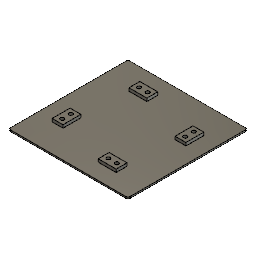
force_plate_bottom (Autodesk Fusion 360 design; units mm, degrees)
Autodesk Fusion 360 part; units mm, degrees
sketch "Sketch1" plane through (0, 0, 0) normal (0, 1, 0) x (1, 0, 0)
  line L0 (-67.5, -70) -> (67.5, -70)
  line L1 (70, -67.5) -> (70, 67.5)
  line L2 (67.5, 70) -> (-67.5, 70)
  line L3 (-70, 67.5) -> (-70, -67.5)
  line L4 (-70, -70) -> (70, 70) construction
  line L5 (70, -70) -> (-70, 70) construction
  arc A0 (-67.5, 70) -> (-70, 67.5) centre (-67.5, 67.5) ccw
  arc A1 (70, 67.5) -> (67.5, 70) centre (67.5, 67.5) ccw
  arc A2 (67.5, -70) -> (70, -67.5) centre (67.5, -67.5) ccw
  arc A3 (-70, -67.5) -> (-67.5, -70) centre (-67.5, -67.5) ccw
  dimension "d1" = 140
  dimension "d2" = 140
  dimension "d25" = 2.5
  dimension "d26" = 2.5
  dimension "d27" = 2.5
  dimension "d28" = 2.5
  constraint horizontal L0
  constraint perpendicular L0 L1
  constraint parallel L0 L2
  constraint parallel L1 L3
  constraint coincident L4 origin
  constraint coincident L5 origin
  constraint coincident L5.end L2
  constraint coincident L5.end L3
  constraint tangent L2 A0
  constraint tangent L3 A0
  constraint coincident L4.end L2
  constraint coincident L4.end L1
  constraint tangent L2 A1
  constraint tangent L1 A1
  constraint coincident L5.start L1
  constraint coincident L5.start L0
  constraint tangent L1 A2
  constraint tangent L0 A2
  constraint coincident L4.start L3
  constraint coincident L4.start L0
  constraint tangent L3 A3
  constraint tangent L0 A3
  measures "d1" distance of L4.end L5.end
  measures "d2" distance of L5.start L4.end
  measures "d25" radius of A0
  measures "d26" radius of A1
  measures "d27" radius of A2
  measures "d28" radius of A3
extrude "Extrude1" add sketch "Sketch1" along normal blind 2
sketch "Sketch11" plane through (0, 0, 0) normal (0, -1, 0) x (1, 0, 0)
  arc A0 (-67.5, 70) -> (-70, 67.5) centre (-67.5, 67.5) ccw
  line L0 (-70, 67.5) -> (-70, -67.5)
  arc A1 (-70, -67.5) -> (-67.5, -70) centre (-67.5, -67.5) ccw
  line L1 (-67.5, -70) -> (67.5, -70)
  arc A2 (67.5, -70) -> (70, -67.5) centre (67.5, -67.5) ccw
  line L2 (70, -67.5) -> (70, 67.5)
  arc A3 (70, 67.5) -> (67.5, 70) centre (67.5, 67.5) ccw
  line L3 (67.5, 70) -> (-67.5, 70)
  line L4 (37.5, 38.65) -> (37.5, 51.35)
  line L5 (-37.5, 51.35) -> (-37.5, 38.65)
  line L6 (-51.35, -37.5) -> (-38.65, -37.5)
  line L7 (-38.65, 37.5) -> (-51.35, 37.5)
  line L8 (37.5, -51.35) -> (37.5, -38.65)
  line L9 (-37.5, -38.65) -> (-37.5, -51.35)
  line L10 (38.65, -37.5) -> (51.35, -37.5)
  line L11 (51.35, 37.5) -> (38.65, 37.5)
  circle A4 centre (-22, -45) radius 2.1
  circle A5 centre (-32, -45) radius 2.1
  circle A6 centre (22, -45) radius 2.1
  circle A7 centre (32, -45) radius 2.1
  circle A8 centre (-45, -22) radius 2.1
  circle A9 centre (-45, -32) radius 2.1
  circle A10 centre (-45, 22) radius 2.1
  circle A11 centre (-45, 32) radius 2.1
  circle A12 centre (-32, 45) radius 2.1
  circle A13 centre (-22, 45) radius 2.1
  circle A14 centre (22, 45) radius 2.1
  circle A15 centre (32, 45) radius 2.1
  circle A16 centre (45, 22) radius 2.1
  circle A17 centre (45, 32) radius 2.1
  circle A18 centre (45, -22) radius 2.1
  circle A19 centre (45, -32) radius 2.1
  line L12 (-51.35, 37.5) -> (-38.65, 37.5)
  line L13 (-38.65, 37.5) -> (-38.65, 16.5)
  line L14 (-38.65, 16.5) -> (-51.35, 16.5)
  line L15 (-51.35, 16.5) -> (-51.35, 37.5)
  line L16 (-51.35, -37.5) -> (-38.65, -37.5)
  line L17 (-38.65, -37.5) -> (-38.65, -16.5)
  line L18 (-38.65, -16.5) -> (-51.35, -16.5)
  line L19 (-51.35, -16.5) -> (-51.35, -37.5)
  line L20 (-37.5, -51.35) -> (-16.5, -51.35)
  line L21 (-16.5, -51.35) -> (-16.5, -38.65)
  line L22 (-16.5, -38.65) -> (-37.5, -38.65)
  line L23 (-37.5, -38.65) -> (-37.5, -51.35)
  line L24 (37.5, -38.65) -> (16.5, -38.65)
  line L25 (16.5, -38.65) -> (16.5, -51.35)
  line L26 (16.5, -51.35) -> (37.5, -51.35)
  line L27 (37.5, -51.35) -> (37.5, -38.65)
  line L28 (38.65, -37.5) -> (51.35, -37.5)
  line L29 (51.35, -37.5) -> (51.35, -16.5)
  line L30 (51.35, -16.5) -> (38.65, -16.5)
  line L31 (38.65, -16.5) -> (38.65, -37.5)
  line L32 (51.35, 37.5) -> (38.65, 37.5)
  line L33 (38.65, 37.5) -> (38.65, 16.5)
  line L34 (38.65, 16.5) -> (51.35, 16.5)
  line L35 (51.35, 16.5) -> (51.35, 37.5)
  line L36 (37.5, 38.65) -> (16.5, 38.65)
  line L37 (16.5, 38.65) -> (16.5, 51.35)
  line L38 (16.5, 51.35) -> (37.5, 51.35)
  line L39 (37.5, 51.35) -> (37.5, 38.65)
  line L40 (-37.5, 38.65) -> (-16.5, 38.65)
  line L41 (-16.5, 38.65) -> (-16.5, 51.35)
  line L42 (-16.5, 51.35) -> (-37.5, 51.35)
  line L43 (-37.5, 51.35) -> (-37.5, 38.65)
  point P0 (0, 45)
  point P1 (-45, 0)
  point P2 (45, 0)
  dimension "d68" = 12.7
  dimension "d73" = 12.7
  dimension "d77" = 4.2
  dimension "d79" = 4.2
  dimension "d81" = 4.2
  dimension "d83" = 4.2
  dimension "d85" = 4.2
  dimension "d87" = 4.2
  dimension "d89" = 4.2
  dimension "d91" = 4.2
  dimension "d93" = 4.2
  dimension "d95" = 4.2
  dimension "d97" = 4.2
  dimension "d99" = 4.2
  dimension "d101" = 4.2
  dimension "d103" = 4.2
  dimension "d105" = 4.2
  dimension "d107" = 4.2
  dimension "d111" = 21
  dimension "d112" = 12.7
  dimension "d113" = 21
  dimension "d114" = 21
  dimension "d115" = 21
  dimension "d116" = 21
  dimension "d117" = 21
  dimension "d118" = 21
  dimension "d119" = 21
  dimension "d120" = 12.7
  constraint parallel L4 L5
  constraint horizontal L6
  constraint parallel L6 L7
  constraint parallel L8 L9
  constraint horizontal L10
  constraint parallel L10 L11
  constraint horizontal L12
  constraint vertical L13
  constraint horizontal L14
  constraint vertical L15
  constraint horizontal L16
  constraint vertical L17
  constraint horizontal L18
  constraint vertical L19
  constraint horizontal L20
  constraint vertical L21
  constraint horizontal L22
  constraint vertical L23
  constraint horizontal L24
  constraint vertical L25
  constraint horizontal L26
  constraint vertical L27
  constraint horizontal L28
  constraint vertical L29
  constraint horizontal L30
  constraint vertical L31
  constraint horizontal L32
  constraint vertical L33
  constraint horizontal L34
  constraint vertical L35
  constraint horizontal L36
  constraint vertical L37
  constraint horizontal L38
  constraint vertical L39
  constraint horizontal L40
  constraint vertical L41
  constraint horizontal L42
  constraint vertical L43
  measures "d68" distance of L7.start L7.end
  measures "d73" distance of L8.start L8.end
  measures "d77" diameter of A4
  measures "d79" diameter of A5
  measures "d81" diameter of A6
  measures "d83" diameter of A7
  measures "d85" diameter of A8
  measures "d87" diameter of A9
  measures "d89" diameter of A10
  measures "d91" diameter of A11
  measures "d93" diameter of A12
  measures "d95" diameter of A13
  measures "d97" diameter of A14
  measures "d99" diameter of A15
  measures "d101" diameter of A16
  measures "d103" diameter of A17
  measures "d105" diameter of A18
  measures "d107" diameter of A19
  measures "d111" distance of L7.end L14.end
  measures "d112" distance of L6.start L6.end
  measures "d113" distance of L6.start L18.end
  measures "d114" distance of L9.end L20.end
  measures "d115" distance of L8.end L24.end
  measures "d116" distance of L10.start L30.end
  measures "d117" distance of L11.start L34.end
  measures "d118" distance of L4.start L36.end
  measures "d119" distance of L5.end L40.end
  measures "d120" distance of L5.end L5.start
extrude "Extrude9" add sketch "Sketch11" along normal blind 3.5 contours L5 L40 L41 L42 L43 | L6 L16 L17 L18 L19 | L8 L24 L25 L26 L27 | L11 L32 L33 L34 L35
hole "Hole4" at (-32, 0, 45) at (-22, 0, 45) at (45, 0, 32) at (45, 0, 22) at (32, 0, -45) at (22, 0, -45) at (-45, 0, -32) at (-45, 0, -22) direction (0, 1, 0) diameter 4.2 depth 5 tip angle 180
move_body "Move2" bodies 1 to x (1, 0, 0) y (0, -1, 0) z (0, 0, -1) at (0, 4, -6.3187)
